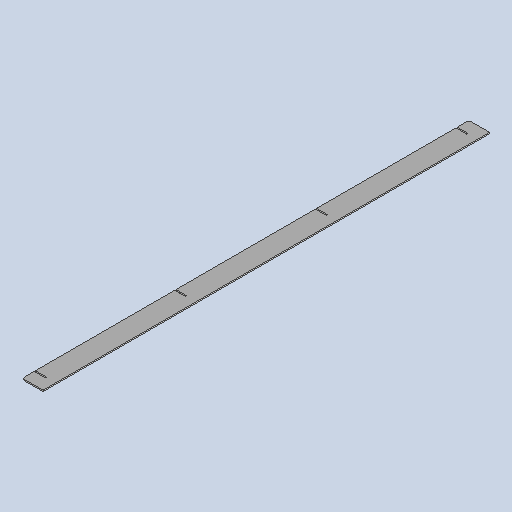
# Autodesk Inventor part: MSC 605 RIB CONE EXIT BACK
Saved by Autodesk Inventor 2025 (Build 290162010, 162A)
## iProperties
Created: 2024-08-26
Part Number: MSC 605 RIB CONE EXIT BACK
Material: Stainless Steel
Document SubType Name: Sheet Metal
Designer: pokla
Density: 8 g/cm^3
Sheet Metal Rule: AISI304 3mm Die 32
Appearance: Default
Stock Number: МОО 605 шпангоут конус выход корма
Mass: 1287.89 g
Surface Area: 1147.13 cm^2
Volume: 160.986 cm^3
Flat Pattern Width: 108 cm
Flat Pattern Length: 5 cm
Flat Pattern Area: 540 cm^2
Sheet Metal Width: 1080,000 mm
Sheet Metal Length: 50,000 mm
Sheet Metal Area: 54000,000 mm^2
Author: pokla
Autodesk Inventor part; units mm, degrees
ref_plane "YZ Plane" through (0, 0, 0) normal (1, 0, 0) x (0, 1, 0)
ref_plane "XZ Plane" through (0, 0, 0) normal (0, 1, 0) x (-1, 0, 0)
ref_plane "XY Plane" through (0, 0, 0) normal (0, 0, 1) x (1, 0, 0)
sketch "Sketch1" plane through (0, 0, 0) normal (0, 0, 1) x (1, 0, 0)
  line L0 (-25, 0) -> (25, 0)
  line L1 (25, 0) -> (25, -1080)
  line L2 (25, -1080) -> (-25, -1080)
  line L3 (-25, -1080) -> (-25, 0)
  point P0 (0, 0)
  point P1 (0, 0)
  point P2 (-25, -1153.2713)
  dimension "d0" = 50
  dimension "d1" = 1080
  measures "d0" distance of L0.start L0.end
  measures "d1" distance of L2.end L0.start
extrude "Plate1" add sketch "Sketch1" along normal mid plane 3
sketch "Sketch2" plane through (0, 0, 1.5) normal (0, 0, 1) x (1, 0, 0)
  line L0 (-25, -708.45) -> (1, -708.45)
  line L1 (1, -708.45) -> (1, -711.55)
  line L2 (1, -711.55) -> (-25, -711.55)
  line L3 (-25, -711.55) -> (-25, -708.45)
  line L4 (-25, -1080) -> (-25, 0) projected
  line L5 (-25, -371.55) -> (1, -371.55)
  line L6 (1, -371.55) -> (1, -368.45)
  line L7 (1, -368.45) -> (-25, -368.45)
  line L8 (-25, -368.45) -> (-25, -371.55)
  line L9 (-25, -1048.45) -> (1, -1048.45)
  line L10 (1, -1048.45) -> (1, -1051.55)
  line L11 (1, -1051.55) -> (-25, -1051.55)
  line L12 (-25, -1051.55) -> (-25, -1048.45)
  line L13 (-25, -31.55) -> (1, -31.55)
  line L14 (1, -31.55) -> (1, -28.45)
  line L15 (1, -28.45) -> (-25, -28.45)
  line L16 (-25, -28.45) -> (-25, -31.55)
  line L17 (-25, -540) -> (1, -540) construction
  point P0 (0, 0)
  point P1 (-25, -710)
  point P2 (-25, -370)
  point P3 (-25, -371.55)
  point P4 (-25, -1050)
  point P5 (-25, -30)
  point P6 (-25, -28.45)
  point P7 (-25, -31.55)
  point P8 (-25, -1048.45)
  point P9 (-25, -1051.55)
  dimension "d16" = 3.1
  dimension "d17" = 26
  dimension "d25" = 340
  dimension "d29" = 340
  dimension "d31" = 340
  constraints: 34 end point, 8 parallel, 6 collinear, 6 midpoint, 5 horizontal, 4 perpendicular, 2 point on line, 2 vertical alignment, 1 other
  measures "d16" distance of L2.end L0.start
  measures "d17" distance of L1.end L2.end
  measures "d25" distance of point (-25, -1050) point (-25, -710)
  measures "d29" distance of point (-25, -30) point (-25, -370)
  measures "d31" distance of point (-25, -710) point (-25, -370)
extrude "Extrusion1" cut sketch "Sketch2" against normal through all
fillet "Corner Round3" radius 6 2 edges at (-25, -1080, 0) (-25, 0, 0)
sketch "Sketch3" plane through (0, 0, -1.5) normal (0, 0, -1) x (-1, 0, 0)
  line L0 (5.4391, -935.4771) -> (-3.5887, -935.4771) construction
  line L1 (-3.5887, -935.4771) -> (-3.5887, -826.531) construction
  line L2 (-3.5887, -826.531) -> (5.4391, -826.531) construction
  line L3 (5.4391, -826.531) -> (5.4391, -935.4771) construction
  point P0 (0, 0)
  dimension "d2" = 3
  dimension "GapSize" = 3
  dimension "SeamGap" = 0.01
  dimension "Thickness" = 3
  dimension "BendRadius" = 5
  dimension "MinimumRemnant" = 6
  dimension "BendReliefDepth" = 1.5
  dimension "BendReliefWidth" = 3
  dimension "CornerReliefSize" = 12
  dimension "JacobiRadiusSize" = 5
  dimension "TransitionRadius" = 5
  constraints: 2 other
mark "Mark1"
equation "\"d2\" = Thickness"
equation "\"d25\" = d31"
equation "\"d29\" = d31"
equation "\"GapSize\" = Thickness"
equation "\"MinimumRemnant\" = 2 * Thickness"
equation "\"BendReliefDepth\" = 0.5 * Thickness"
equation "\"BendReliefWidth\" = Thickness"
equation "\"CornerReliefSize\" = 4 * Thickness"
equation "\"JacobiRadiusSize\" = BendRadius"
equation "\"TransitionRadius\" = BendRadius"
body "Solid1"
